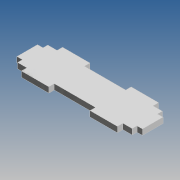
# Autodesk Inventor part: CaissonCoteBiais
Saved by Autodesk Inventor 2019 (Build 230136000, 136)
## iProperties
Created: 2019-08-26
Part Number: CaissonCoteBiais
Material: PVC-U
Document SubType Name: Modeling
Designer: jeremias.salamin
Density: 1.4 g/cm^3
Appearance: Lisse - Blanc
Description: CaissonCôtéBiais
Author: jeremias.salamin
Autodesk Inventor part; units mm, degrees
ref_plane "YZ Plane" through (0, 0, 0) normal (1, 0, 0) x (0, 1, 0)
ref_plane "XZ Plane" through (0, 0, 0) normal (0, 1, 0) x (-1, 0, 0)
ref_plane "XY Plane" through (0, 0, 0) normal (0, 0, 1) x (1, 0, 0)
sketch "Sketch1" plane through (0, 0, 0) normal (0, 0, 1) x (1, 0, 0)
  line L0 (0, 6.16) -> (0, -6.16) construction
  line L1 (-23.38, 0) -> (23.38, 0) construction
  line L2 (16.7, -4.4) -> (-16.7, -4.4)
  line L3 (-16.7, -4.4) -> (-16.7, 4.4)
  line L4 (-16.7, 4.4) -> (16.7, 4.4)
  line L5 (16.7, 4.4) -> (16.7, -4.4)
  line L6 (16.7, -4.4) -> (-16.7, 4.4) construction
  line L7 (-16.7, -4.4) -> (16.7, 4.4) construction
  point P0 (0, 0)
  dimension "d0" = 33.4
  dimension "d1" = 8.8
  constraints: 12 end point, 2 midpoint, 2 parallel, 1 horizontal, 1 perpendicular
  measures "d0" distance of L3.end L4.end
  measures "d1" distance of L2.end L3.end
extrude "Extrusion1" add sketch "Sketch1" along normal mid plane 1.6
sketch "Esquisse2" plane through (0, 0, 0.8) normal (0, 0, 1) x (1, 0, 0)
  line L0 (-16.7, -4.4) -> (16.7, -4.4) construction
  line L1 (16.7, -4.4) -> (16.7, 4.4) construction
  line L2 (16.7, 4.4) -> (-16.7, 4.4) construction
  line L3 (-16.7, 4.4) -> (-16.7, -4.4) construction
  line L4 (0, 8.08) -> (0, -6.48) construction
  line L5 (-23.38, 0) -> (23.38, 0) construction
  line L6 (-14, 4.4) -> (-6, 4.4)
  line L7 (-6, 4.4) -> (-6, 6)
  line L8 (-6, 6) -> (-14, 6)
  line L9 (-14, 6) -> (-14, 4.4)
  line L10 (6, 4.4) -> (14, 4.4)
  line L11 (14, 4.4) -> (14, 6)
  line L12 (14, 6) -> (6, 6)
  line L13 (6, 6) -> (6, 4.4)
  point P0 (0, 0)
  dimension "d4" = 8
  dimension "d5" = 1.6
  dimension "d8" = 20
  constraints: 16 end point, 2 horizontal, 2 parallel, 1 perpendicular, 1 point on line, 9 other
  measures "d4" distance of L8.end L7.end
  measures "d5" distance of L7.end L6.end
  measures "d8" distance of L6.start L10.start
extrude "Extrusion2" add sketch "Esquisse2" against normal blind 1.6
mirror "Symétrie1" about plane through (0, 0, 0) normal (0, 1, 0) of "Extrusion2"
sketch "Esquisse3" plane through (0, 0, 0.8) normal (0, 0, 1) x (1, 0, 0)
  line L0 (-16.7, -4.4) -> (-14, -4.4) construction
  line L1 (-14, -6) -> (-14, -4.4) construction
  line L2 (-6, -6) -> (-14, -6) construction
  line L3 (-6, -4.4) -> (-6, -6) construction
  line L4 (-6, -4.4) -> (6, -4.4) construction
  line L5 (6, -6) -> (6, -4.4) construction
  line L6 (14, -6) -> (6, -6) construction
  line L7 (14, -4.4) -> (14, -6) construction
  line L8 (14, -4.4) -> (16.7, -4.4) construction
  line L9 (16.7, -4.4) -> (16.7, 4.4) construction
  line L10 (16.7, 4.4) -> (14, 4.4) construction
  line L11 (14, 4.4) -> (14, 6) construction
  line L12 (14, 6) -> (6, 6) construction
  line L13 (6, 6) -> (6, 4.4) construction
  line L14 (6, 4.4) -> (-6, 4.4) construction
  line L15 (-6, 4.4) -> (-6, 6) construction
  line L16 (-6, 6) -> (-14, 6) construction
  line L17 (-14, 6) -> (-14, 4.4) construction
  line L18 (-14, 4.4) -> (-16.7, 4.4) construction
  line L19 (-16.7, 4.4) -> (-16.7, -4.4) construction
  line L20 (-23.38, 0) -> (23.38, 0) construction
  line L21 (0, 8.4) -> (0, -8.4) construction
  line L22 (-16.7, 3) -> (-18.3, 3)
  line L23 (-18.3, 3) -> (-18.3, -3)
  line L24 (-18.3, -3) -> (-16.7, -3)
  line L25 (-16.7, -3) -> (-16.7, 3)
  line L26 (16.7, 3) -> (18.3, 3)
  line L27 (18.3, 3) -> (18.3, -3)
  line L28 (18.3, -3) -> (16.7, -3)
  line L29 (16.7, -3) -> (16.7, 3)
  point P0 (0, 0)
  dimension "d15" = 1.6
  dimension "d16" = 6
  constraints: 16 end point, 4 symmetric about line, 2 parallel, 1 horizontal, 1 perpendicular, 1 point on line, 1 other
  measures "d15" distance of L23.end L24.end
  measures "d16" distance of L22.end L23.end
extrude "Extrusion3" add sketch "Esquisse3" against normal blind 1.6
